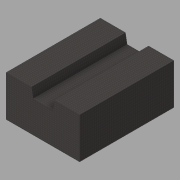
# Autodesk Inventor part: FerrisWheelCarriageKGR
Saved by Autodesk Inventor 2018 (Build 220112000, 112)
## iProperties
Created: 2018-01-20
Part Number: FerrisWheelCarriageKGR
Material: Concrete
Document SubType Name: Modeling
Designer: Emperor Gai
Density: 2.40731 g/cm^3
Appearance: Exposed Aggregate - Coarse
Author: Emperor Gai
Autodesk Inventor part; units mm, degrees
ref_plane "YZ Plane" through (0, 0, 0) normal (1, 0, 0) x (0, 1, 0)
ref_plane "XZ Plane" through (0, 0, 0) normal (0, 1, 0) x (-1, 0, 0)
ref_plane "XY Plane" through (0, 0, 0) normal (0, 0, 1) x (1, 0, 0)
sketch "Sketch1" plane through (0, 0, 0) normal (0, 0, 1) x (1, 0, 0)
  line L0 (-3564.8334, 914.4) -> (-3564.8334, -3048)
  line L1 (-3564.8334, -3048) -> (3564.8334, -3048)
  line L2 (3564.8334, -3048) -> (3564.8334, 914.4)
  line L3 (3564.8334, 914.4) -> (1126.4334, 914.4)
  line L4 (1126.4334, 914.4) -> (965.2, 0)
  line L5 (965.2, 0) -> (-965.2, 0)
  line L6 (-965.2, 0) -> (-1126.4334, 914.4)
  line L7 (-1126.4334, 914.4) -> (-3564.8334, 914.4)
  point P0 (0, 0)
  point P1 (0, 0)
  dimension "d0" = 2438.4
  dimension "d1" = 1930.4
  dimension "d2" = 914.4
  dimension "d3" = 100
  dimension "d4" = 100
  dimension "d5" = 3048
  constraints: 16 end point, 4 parallel, 2 collinear, 1 coincident, 1 horizontal, 1 midpoint, 1 vertical
  measures "d0" distance of L6.end L0.start
  measures "d1" distance of L4.end L5.end
  measures "d2" distance between parallel lines of L5 L7
  measures "d3" angle of L5 L6
  measures "d4" angle of L5 L4
  measures "d5" distance between parallel lines of L5 L1
extrude "Extrusion1" add sketch "Sketch1" along normal mid plane 9144
equation "\"d4\" = d3"
body "Solid1"
